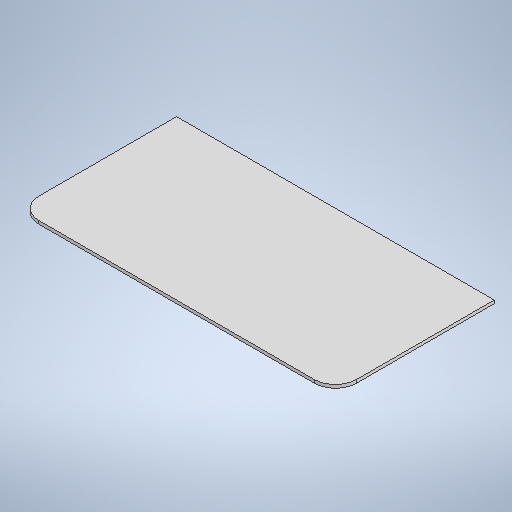
# Autodesk Inventor part: Chassis Top Plate
Saved by Autodesk Inventor 2025.2 (Build 292293000, 293)
## iProperties
Created: 2025-01-24
Part Number: Chassis Top Plate
Material: Generic
Document SubType Name: Modeling
Designer: Matt Tidd
Density: 1 g/cm^3
Appearance: Default
Author: Matt Tidd
Autodesk Inventor part; units mm, degrees
ref_plane "YZ Plane" through (0, 0, 0) normal (1, 0, 0) x (0, 1, 0)
ref_plane "XZ Plane" through (0, 0, 0) normal (0, 1, 0) x (-1, 0, 0)
ref_plane "XY Plane" through (0, 0, 0) normal (0, 0, 1) x (1, 0, 0)
sketch "Sketch1" plane through (0, 0, 0) normal (0, 1, 0) x (-1, 0, 0)
  line L0 (20, 0) -> (280, 0)
  line L1 (300, -20) -> (300, -150)
  line L2 (300, -150) -> (0, -150)
  line L3 (0, -150) -> (0, -20)
  arc A0 (300, -20) -> (280, 0) centre (280, -20) ccw
  arc A1 (20, 0) -> (0, -20) centre (20, -20) ccw
  line L4 (300, -150) -> (0, -150)
  line L5 (0, -150) -> (0, -207)
  line L6 (0, -207) -> (300, -207)
  line L7 (300, -207) -> (300, -150)
  point P0 (0, 0)
  point P1 (300, 0)
  dimension "d0" = 300
  dimension "d1" = 150
  dimension "d2" = 20
  dimension "d5" = 57
  constraints: 16 end point, 4 parallel, 4 point on circle, 4 point on line, 4 tangent, 2 centre point, 2 horizontal, 2 perpendicular, 1 equal radius
  measures "d0" distance of L1.end L2.end
  measures "d1" distance of point (300, 0) L1.end
  measures "d2" radius of A0
  measures "d5" distance of L5.end L4.end
extrude "Extrusion1" add sketch "Sketch1" along normal blind 3 contours L0 A0 L1 L2 L3 A1
body "Solid1"
